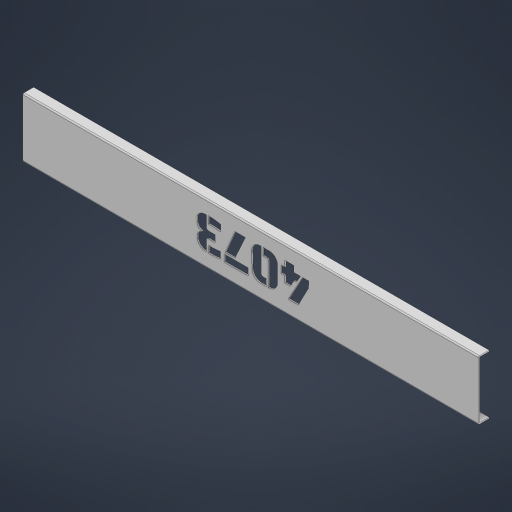
# Autodesk Inventor part: Chassis FrontandBack
Saved by Autodesk Inventor 2023 (Build 270158000, 158)
## iProperties
Created: 2022-04-13
Part Number: Chassis FrontandBack
Material: Generic
Document SubType Name: Modeling
Designer: timmy
Density: 1 g/cm^3
Appearance: Default
Author: timmy
Autodesk Inventor part; units mm, degrees
ref_plane "YZ Plane" through (0, 0, 0) normal (1, 0, 0) x (0, 1, 0)
ref_plane "XZ Plane" through (0, 0, 0) normal (0, 1, 0) x (-1, 0, 0)
ref_plane "XY Plane" through (0, 0, 0) normal (0, 0, 1) x (1, 0, 0)
sketch "Sketch1" plane through (0, 0, 0) normal (0, 0, 1) x (1, 0, 0)
  line L0 (0, 0) -> (609.6, 0)
  line L1 (609.6, 0) -> (609.6, 76.2)
  line L2 (609.6, 76.2) -> (0, 76.2)
  line L3 (0, 76.2) -> (0, 0)
  dimension "d0" = 609.6
  dimension "d1" = 76.2
  constraints: 8 end point, 2 parallel, 1 horizontal, 1 perpendicular
  measures "d0" distance of L2.end L1.end
  measures "d1" distance of L1.end L0.end
extrude "Extrusion1" add sketch "Sketch1" along normal blind 1.5875
sketch "Sketch2" plane through (0, 76.2, 0) normal (0, 1, 0) x (1, 0, 0)
  line L0 (609.6, 0) -> (0, 0) projected
  line L1 (0, 0) -> (0, -1.5875) projected
  line L2 (609.6, -1.5875) -> (0, -1.5875) projected
  line L3 (609.6, 0) -> (609.6, -1.5875) projected
  line L4 (609.6, -1.5875) -> (0, -1.5875)
  line L5 (0, -1.5875) -> (0, 12.7)
  line L6 (0, 12.7) -> (609.6, 12.7)
  line L7 (609.6, 12.7) -> (609.6, -1.5875)
  dimension "d39" = 12.7
  constraints: 8 end point, 2 parallel, 1 horizontal, 1 perpendicular
  measures "d39" distance between parallel lines of L6 L0
extrude "Extrusion2" add sketch "Sketch2" along normal blind 1.5875
fillet "Fillet1" radius 1.5875 1 edges at (304.8, 77.7875, 1.5875)
sketch "Sketch3" plane through (0, 0, 0) normal (0, -1, 0) x (1, 0, 0)
  line L0 (609.6, 0) -> (0, 0) projected
  line L1 (0, -12.7) -> (0, 0) projected
  line L2 (609.6, -12.7) -> (0, -12.7) projected
  line L3 (609.6, 0) -> (609.6, -12.7) projected
extrude "Extrusion3" add sketch "Sketch3" along normal blind 1.5875
sketch "Sketch4" plane through (0, 76.2, -12.7) normal (-1, 0, 0) x (0, 0, 1)
  line L0 (12.7, -76.2) -> (0, -76.2) projected
  line L1 (0, -76.2) -> (0, -77.7875) projected
  line L2 (12.7, -77.7875) -> (0, -77.7875) projected
  line L3 (12.7, -76.2) -> (12.7, -77.7875) projected
  arc A0 (14.2875, 0) -> (12.7, 1.5875) centre (12.7, 0) ccw projected
  line L4 (0, 1.5875) -> (12.7, 1.5875) projected
  line L5 (0, 0) -> (0, 1.5875) projected
  line L6 (0, 0) -> (12.7, 0) projected
  line L7 (12.7, 0) -> (12.7, -76.2) projected
  line L8 (12.7, -76.2) -> (14.2875, -76.2) projected
  line L9 (14.2875, -76.2) -> (14.2875, 0) projected
  line L10 (12.7, -76.2) -> (14.2875, -76.2)
  line L11 (14.2875, -76.2) -> (14.2875, -77.7875)
  line L12 (14.2875, -77.7875) -> (12.7, -77.7875)
  line L13 (12.7, -77.7875) -> (12.7, -76.2)
  constraints: 8 end point, 2 parallel, 1 horizontal, 1 perpendicular
extrude "Extrusion4" add sketch "Sketch4" against normal up to surface (609.6 mm away) contours L8 L11 L12 L3
fillet "Fillet2" radius 1.5875 1 edges at (304.8, -1.5875, 1.5875)
sketch "Sketch5" plane through (0, 0, 1.5875) normal (0, 0, 1) x (1, 0, 0)
  line L0 (391.8077, 9.2075) -> (217.7923, 9.2075) construction
  line L1 (217.7923, 9.2075) -> (217.7923, 67.0009) construction
  line L2 (217.7923, 67.0009) -> (391.8077, 67.0009) construction
  line L3 (391.8077, 67.0009) -> (391.8077, 9.2075) construction
  line L4 (368.7246, 16.9668) -> (355.2902, 16.9668)
  line L5 (355.2902, 16.9668) -> (374.313, 51.6075)
  line L6 (366.0229, 42.0591) -> (362.766, 42.0591)
  line L7 (362.766, 42.0591) -> (358.2013, 33.4623)
  line L8 (358.2013, 33.4623) -> (350.738, 33.4623)
  line L9 (345.5567, 42.0591) -> (345.5567, 51.6075)
  line L10 (345.5567, 51.6075) -> (350.738, 51.6075)
  line L11 (350.738, 51.6075) -> (350.738, 59.6755)
  line L12 (350.738, 59.6755) -> (362.766, 59.6755)
  line L13 (362.766, 59.6755) -> (362.766, 51.6075)
  line L14 (362.766, 51.6075) -> (371.6483, 51.6075)
  line L15 (371.6483, 51.6075) -> (366.0229, 42.0591)
  line L16 (283.8325, 28.8388) -> (297.8915, 59.6755)
  line L17 (283.8325, 59.6755) -> (270.9618, 28.8388)
  line L18 (270.9618, 28.8388) -> (283.8325, 28.8388)
  line L19 (301.3907, 16.9668) -> (301.3907, 26.3815)
  line L20 (301.3907, 26.3815) -> (269.4747, 26.3815)
  line L21 (301.3907, 16.9668) -> (269.4747, 16.9668)
  line L22 (328.4185, 16.8456) -> (328.4185, 47.9611)
  line L23 (321.4042, 50.2314) -> (321.4042, 60.0732)
  line L24 (340.8479, 47.9611) -> (340.8479, 28.9034)
  arc A0 (328.4185, 47.9611) -> (326.7126, 50.2314) centre (326.1181, 48.0086) ccw
  arc A1 (328.4185, 16.8456) -> (340.8479, 28.9034) centre (328.8598, 28.8258) ccw
  line L25 (318.8829, 60.0719) -> (318.8829, 29.6859)
  line L26 (325.6836, 26.3815) -> (325.6836, 16.781)
  line L27 (325.6836, 16.781) -> (319.4882, 16.781)
  arc A2 (306.7329, 27.5963) -> (319.4882, 16.781) centre (318.2151, 28.2088) ccw
  line L28 (306.7329, 27.5963) -> (306.252, 48.615)
  arc A3 (318.8829, 60.0719) -> (306.252, 48.615) centre (317.5294, 48.873) ccw
  line L29 (321.4042, 60.0732) -> (328.4185, 60.0732)
  arc A4 (340.8479, 47.9611) -> (328.4185, 60.0732) centre (329.7877, 49.0447) ccw
  line L30 (609.6, 0) -> (609.6, 76.2) projected
  line L31 (0, 0) -> (0, 76.2) projected
  line L32 (609.6, 0) -> (0, 0) projected
  line L33 (0, 76.2) -> (609.6, 76.2) projected
  line L34 (297.8915, 59.6755) -> (283.8325, 59.6755)
  line L35 (269.4747, 26.3815) -> (269.4747, 16.9668)
  line L36 (326.7126, 50.2314) -> (321.4042, 50.2314)
  line L37 (368.7246, 16.9668) -> (382.3802, 43.1657)
  line L38 (382.3802, 43.1657) -> (382.5469, 51.6075)
  line L39 (382.5469, 51.6075) -> (374.313, 51.6075)
  line L40 (345.5567, 42.0591) -> (350.738, 42.0591)
  line L41 (350.738, 42.0591) -> (350.738, 33.4623)
  arc A5 (318.8829, 29.6859) -> (321.6099, 25.999) centre (321.7802, 28.9769) ccw
  arc A6 (321.6099, 25.999) -> (325.6836, 26.3815) centre (322.9641, 33.4611) ccw
  line L42 (257.2547, 33.4734) -> (257.2547, 42.6715)
  line L43 (257.2547, 42.6715) -> (247.6149, 42.6715)
  line L44 (245.5572, 46.0253) -> (245.5572, 59.7083)
  line L45 (233.0099, 52.0098) -> (233.0099, 45.4817)
  line L46 (240.4004, 38.1857) -> (240.4004, 37.57)
  line L47 (233.3728, 30.9594) -> (233.3728, 25.8822)
  line L48 (245.5572, 16.9419) -> (245.7765, 30.5952)
  arc A7 (233.3728, 25.8822) -> (245.5572, 16.9419) centre (245.0741, 29.0566) ccw
  arc A8 (240.4004, 37.57) -> (233.3728, 30.9594) centre (241.8707, 28.9661) ccw
  arc A9 (233.0099, 45.4817) -> (240.4004, 38.1857) centre (240.5679, 45.7465) ccw
  line L49 (257.2547, 33.4734) -> (248.2741, 33.4734)
  arc A10 (248.2741, 33.4734) -> (245.7765, 30.5952) centre (248.2741, 30.9507) ccw
  arc A11 (245.5572, 46.0253) -> (247.6149, 42.6715) centre (248.5719, 45.5669) ccw
  arc A12 (245.5572, 59.7083) -> (233.0099, 52.0098) centre (243.9929, 48.1836) ccw
  line L50 (264.4301, 17.9919) -> (264.4301, 26.8729)
  arc A13 (254.6467, 16.781) -> (264.4301, 17.9919) centre (253.1662, 68.8681) ccw
  line L51 (248.5719, 25.999) -> (248.5719, 16.781)
  line L52 (248.5719, 16.781) -> (254.6467, 16.781)
  arc A14 (248.5719, 25.999) -> (264.4301, 26.8729) centre (252.074, 106.7711) ccw
  arc A15 (264.6926, 49.5598) -> (248.2741, 50.5346) centre (251.6559, -31.2579) ccw
  line L53 (248.2741, 50.5346) -> (248.0544, 60.0732)
  line L54 (248.0544, 60.0732) -> (252.074, 60.1658)
  line L55 (264.6926, 49.5598) -> (264.6926, 58.3373)
  arc A16 (264.6926, 58.3373) -> (252.074, 60.1658) centre (243.9281, -40.5085) ccw
  point P0 (0, 38.1)
  point P1 (217.7923, 38.1042)
  constraints: 96 end point, 34 point on circle, 17 centre point, 12 horizontal, 10 vertical, 7 perpendicular, 4 parallel, 4 point on line, 2 midpoint, 2 tangent, 2 other
extrude "Extrusion9" cut sketch "Sketch5" against normal blind 25.4 contours L4 L5 L39 L38 L37 | L6 L7 L8 L41 L40 L9 L10 L11 L12 L13 L14 L15 | L18 L17 L34 L16 | L21 L35 L20 L19 | L22 A0 L36 L23 L29 A4 L24 A1 | L25 A5 A6 L26 L27 A2 L28 A3 | L49 A10 L48 A7 L47 A8 L46 A9 L45 A12 L44 A11 L43 L42 | A13 L52 L51 A14 L50 | A15 L53 L54 A16 L55
body "Solid1"
